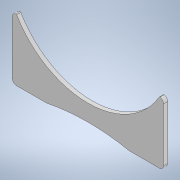
# Autodesk Inventor part: Montage_Fuss
Saved by Autodesk Inventor 2022.2 (Build 262287010, 287A)
## iProperties
Created: 2024-01-10
Part Number: Montage_Fuss
Material: Generisch
Document SubType Name: Modeling
Designer: ppovolni
Density: 1 g/cm^3
Appearance: Vorgabe
Author: ppovolni
Autodesk Inventor part; units mm, degrees
ref_plane "YZ Plane" through (0, 0, 0) normal (1, 0, 0) x (0, 1, 0)
ref_plane "XZ Plane" through (0, 0, 0) normal (0, 1, 0) x (-1, 0, 0)
ref_plane "XY Plane" through (0, 0, 0) normal (0, 0, 1) x (1, 0, 0)
sketch "Skizze1" plane through (0, 0, 0) normal (0, 0, 1) x (1, 0, 0)
  circle A0 centre (0, 0) radius 100 construction
  arc A1 (-86.2926, -50.5331) -> (86.2926, -50.5331) centre (0, 0) ccw
  line L0 (-86.6025, -50) -> (0, 0) construction
  line L1 (0, 0) -> (86.6025, -50) construction
  line L2 (0, -467) -> (0, 194.5) construction
  line L3 (-86.6025, -125) -> (86.6025, -125)
  line L4 (-86.6025, -50) -> (-86.6025, -50)
  line L5 (-91.6025, -55) -> (-91.6025, -120)
  line L6 (86.6025, -50) -> (86.6025, -50)
  line L7 (91.6025, -55) -> (91.6025, -120)
  arc A2 (-87.2937, -50.048) -> (-91.6025, -55) centre (-86.6025, -55) ccw
  arc A3 (91.6025, -55) -> (87.2937, -50.048) centre (86.6025, -55) ccw
  arc A4 (-86.2926, -50.5331) -> (-87.2937, -50.048) centre (-87.1555, -51.0384) ccw
  arc A5 (87.2937, -50.048) -> (86.2926, -50.5331) centre (87.1555, -51.0384) ccw
  arc A6 (-91.6025, -120) -> (-86.6025, -125) centre (-86.6025, -120) ccw
  arc A7 (86.6025, -125) -> (91.6025, -120) centre (86.6025, -120) ccw
  arc A8 (50, -125) -> (-50, -125) centre (0, -372.5) ccw
  point P0 (0, -100)
  point P1 (-91.6025, -50)
  point P2 (0, -125)
  point P3 (0, -120)
  dimension "d0" = 200
  dimension "d1" = 60
  dimension "d2" = 5
  dimension "d3" = 25
  dimension "d4" = 5
  dimension "d5" = 1
  dimension "d6" = 5
  dimension "d7" = 50
  dimension "d8" = 50
  dimension "d9" = 5
  constraints: 24 point on circle, 14 end point, 12 tangent, 9 centre point, 4 equal radius, 4 point on line, 3 horizontal, 2 coincident, 2 vertical, 1 midpoint, 1 vertical alignment
  measures "d0" diameter of A0
  measures "d1" angle of L2 L0
  measures "d2" distance of L0.start point (-91.603, -50)
  measures "d3" distance from line of L3 point (0, -100)
  measures "d4" radius of A2
  measures "d5" radius of A4
  measures "d6" radius of A6
  measures "d7" distance of A8.start point (0, -125)
  measures "d8" distance of A8.end point (0, -125)
  measures "d9" distance of point (0, -125) point (0, -120)
extrude "Extrusion1" add sketch "Skizze1" along normal blind 5 contours A1 A5 A3 L7 A7 L3 A8 A6 L5 A2 A4
